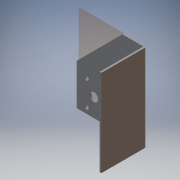
# Autodesk Inventor part: base
Saved by Autodesk Inventor 2019 (Build 230136000, 136)
## iProperties
Created: 2020-04-04
Part Number: base
Material: Generic
Document SubType Name: Modeling
Designer: Hermann
Density: 1 g/cm^3
Appearance: Default
Author: Hermann
Autodesk Inventor part; units mm, degrees
ref_plane "YZ Plane" through (0, 0, 0) normal (1, 0, 0) x (0, 1, 0)
ref_plane "XZ Plane" through (0, 0, 0) normal (0, 1, 0) x (-1, 0, 0)
ref_plane "XY Plane" through (0, 0, 0) normal (0, 0, 1) x (1, 0, 0)
sketch "Sketch1" plane through (0, 0, 0) normal (0, 1, 0) x (-1, 0, 0)
  line L0 (120, 0) -> (5, 0)
  line L1 (0, 5) -> (0, 80)
  arc A0 (0, 5) -> (5, 0) centre (5, 5) ccw
  point P0 (0, 0)
  dimension "d0" = 120
  dimension "d1" = 80
  dimension "d2" = 5
  constraints: 4 end point, 2 point on circle, 2 point on line, 2 tangent, 1 centre point, 1 horizontal, 1 perpendicular
  measures "d0" distance of L0.start point (0, 0)
  measures "d1" distance of point (0, 0) L1.end
  measures "d2" radius of A0
surface extrude "ExtrusionSrf1" sketch "Sketch1" along normal blind 150 and the other way blind 2 shown yes curves L1 A0 L0
thicken "Thicken1" operation new thickness 3.2 both sides no extend neighbours no toward (0, 0, 1) faces at (-43.3333, 48.6667, 0) (-2.5, 99.3333, 0.6699) (0, 48.6667, 55)
sketch "Sketch2" plane through (-5, -2, 0) normal (0, 0, -1) x (-1, 0, 0)
  point P0 (-5, 2)
  point P1 (85, 32)
  dimension "d16" = 30
  dimension "d17" = 90
  measures "d16" vertical distance of point (-5, 2) point (85, 32)
  measures "d17" horizontal distance of point (-5, 2) point (85, 32)
hole "Hole1" at (-90, 30, 0) direction (0, 0, 1) diameter 15 depth 22.2 tip angle 118
sketch "Sketch3" plane through (-120, -2, 3.2) normal (0, 0, 1) x (1, 0, 0)
  circle A0 centre (30, 32) radius 25.4
  circle A1 centre (30, 32) radius 7.5 projected
  line L0 (30, 32) -> (92.1699, 32)
  line L1 (30, 32) -> (-1.9104, -23.2704)
  line L2 (30, 32) -> (3.6048, 77.7179)
  point P0 (120, 2)
  point P1 (17.3, 53.997)
  point P2 (17.3, 10.003)
  point P3 (55.4, 32)
  dimension "d25" = 0
  dimension "d26" = 0
  dimension "d27" = 50.8
  dimension "d28" = 120
  dimension "d29" = 120
  constraints: 6 end point, 3 point on circle, 3 point on line, 1 centre point, 1 horizontal
  measures "d25" distance of L0.start A0.centre
  measures "d26" distance of L0.start A0.centre
  measures "d27" diameter of A0
  measures "d28" angle of L0 L2
  measures "d29" angle of L0 L1
hole "Hole2" at (-102.7, 51.997, 3.2) at (-102.7, 8.003, 3.2) at (-64.6, 30, 3.2) direction (0, 0, -1) diameter 7 depth 22.2 tip angle 118
chamfer "Chamfer1" distance 80 angle 45 1 edges at (-120, 150, 1.6)
body "Solid1"
body "Srf1"
